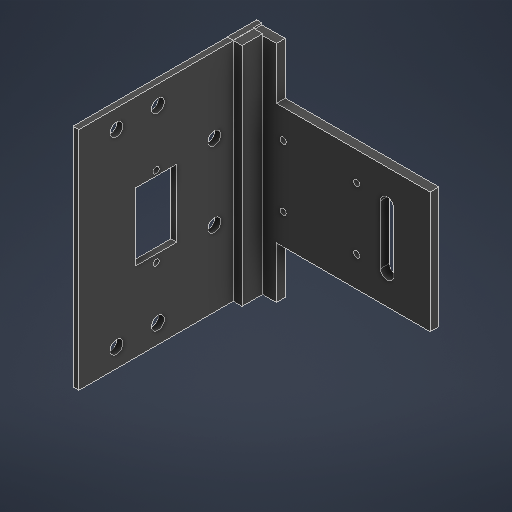
# Autodesk Inventor part: cameramount
Saved by Autodesk Inventor 2027 (Build 310192000, 192)
## iProperties
Created: 2026-06-30
Part Number: cameramount
Material: Generic
Document SubType Name: Modeling
Designer: uchiha
Density: 1 g/cm^3
Appearance: Default
Author: uchiha
Autodesk Inventor part; units mm, degrees
sketch "Sketch1" plane through (0, 0, 0) normal (1, 0, 0) x (0, 1, 0)
  circle A0 centre (-12.8712, -19.8017) radius 2.1703
  circle A1 centre (-32.0775, -0.5955) radius 2.1703
  circle A2 centre (31.9433, -0.5955) radius 2.1703
  circle A3 centre (31.9433, 13.4891) radius 2.1703
  circle A4 centre (-32.0775, 13.4891) radius 2.1703
  circle A5 centre (12.7371, -19.8017) radius 2.1703
  line L0 (38.3454, 26.2933) -> (38.3454, -26.2038)
  line L1 (-38.4796, 26.2933) -> (38.3454, 26.2933)
  line L2 (-38.4796, 26.2933) -> (-38.4796, -26.2038)
  line L3 (38.3454, -26.2038) -> (-38.4796, -26.2038)
  circle A6 centre (-32.0775, 13.4891) radius 2.1703
  circle A7 centre (-32.0775, -0.5955) radius 2.1703
  line L4 (11.5, -7) -> (-11.5, -7)
  line L5 (-11.5, -7) -> (-11.5, 7)
  line L6 (-11.5, 7) -> (11.5, 7)
  line L7 (11.5, 7) -> (11.5, -7)
  line L8 (11.5, -7) -> (-11.5, 7) construction
  line L9 (-11.5, -7) -> (11.5, 7) construction
  circle A8 centre (13.2, 0) radius 1
  circle A9 centre (-14, 0) radius 1
  point P0 (0, 0)
  point P1 (-11.5, 0)
  dimension "d26" = 23
  dimension "d27" = 14
  dimension "d28" = 27.2
  dimension "d29" = 2
  dimension "d30" = 2.5
  constraints: 20 end point, 10 centre point, 3 midpoint, 2 parallel, 1 equal radius, 1 horizontal, 1 perpendicular
  measures "d26" distance of L5.end L6.end
  measures "d27" distance of L4.end L5.end
  measures "d28" distance of A8.centre A9.centre
  measures "d29" diameter of A8
  measures "d30" distance of point (-11.5, 0) A9.centre
ref_plane "Work Plane6" through (0, -38.4796, -26.2038) normal (0, 0, -1) x (-1, 0, 0)
sketch "Sketch3" plane through (0, -38.4796, -26.2038) normal (0, 0, -1) x (-1, 0, 0)
  line L0 (0, 76.825) -> (-3, 76.825) projected
  line L1 (0, 0) -> (-3, 0) projected
  line L2 (-3, 76.825) -> (0, 76.825)
  line L3 (0, 76.825) -> (0, 0)
  line L4 (0, 0) -> (-3, 0)
  line L5 (-3, 0) -> (-3, 76.825)
  line L6 (0, 0) -> (0, 76.825) projected
  line L7 (-3, 0) -> (-3, 76.825) projected
  line L8 (0.01, -0.01) -> (0.01, 76.835)
  line L9 (0.01, 76.835) -> (-3.01, 76.835)
  line L10 (-3.01, 76.835) -> (-3.01, -0.01)
  line L11 (-3.01, -0.01) -> (0.01, -0.01)
  point P0 (0, 38.4796)
  dimension "d3" = 0.01
  constraints: 16 end point, 4 parallel, 2 perpendicular, 1 horizontal, 3 other
  measures "d3" distance between parallel lines of L3 L8
extrude "Extrusion2" add sketch "Sketch3" along normal blind 10 contours L3 L1 L5 L0
ref_plane "Work Plane3" through (0, 0, 0) normal (-1, 0, 0) x (0, 0, 1)
sketch "Sketch4" plane through (0, 0, 0) normal (-1, 0, 0) x (0, 0, 1)
  line L0 (26.2933, -38.4796) -> (-36.2038, -38.4796) projected
  line L1 (-36.2038, 38.422) -> (-33.2038, 38.422)
  line L2 (-33.2038, 38.422) -> (-33.2038, -38.4796)
  line L3 (-33.2038, -38.4796) -> (-36.2038, -38.4796)
  line L4 (-36.2038, -38.4796) -> (-36.2038, 38.422)
  line L5 (-36.2038, 38.3454) -> (-36.2038, -38.4796) projected
  point P0 (0, 0)
  dimension "d8" = 3
  constraints: 8 end point, 2 parallel, 1 collinear, 1 horizontal, 1 perpendicular, 1 point on line
  measures "d8" distance between parallel lines of L4 L2
extrude "Extrusion3" add sketch "Sketch4" against normal blind 60
ref_plane "Work Plane1" through (0, -38.4796, -36.2038) normal (0, 0, -1) x (-1, 0, 0)
ref_plane "Work Plane4" through (0, -38.4796, -36.2038) normal (0, 0, -1) x (-1, 0, 0)
sketch "Sketch6" plane through (0, -38.4796, -36.2038) normal (0, 0, -1) x (-1, 0, 0)
  line L0 (0, 38.4796) -> (-60, 38.4508)
  line L1 (-60, 0) -> (-60, 76.9016) projected
  line L2 (-30, 76.2766) -> (-30, 0)
  line L3 (-43.0944, 47.6588) -> (-43.0944, 27.6588)
  arc A0 (-47.5944, 27.6588) -> (-43.0944, 27.6588) centre (-45.3444, 27.6588) ccw
  line L4 (-47.5944, 27.6588) -> (-47.5944, 47.6588)
  arc A1 (-43.0944, 47.6588) -> (-47.5944, 47.6588) centre (-45.3444, 47.6588) ccw
  circle A2 centre (-35, 27.8243) radius 1
  circle A3 centre (-10, 27.8243) radius 1
  circle A4 centre (-35, 48.8243) radius 1
  circle A5 centre (-10, 48.8243) radius 1
  line L5 (-57.8444, 58.6588) -> (-57.8444, 17.5214)
  line L6 (-57.8444, 17.5214) -> (-2.3444, 17.5214)
  line L7 (-2.3444, 17.5214) -> (-2.3444, 58.6588)
  line L8 (-2.3444, 58.6588) -> (-57.8444, 58.6588)
  line L9 (-57.8444, 58.6588) -> (-60, 58.6588)
  line L10 (-2.3444, 58.6588) -> (0, 58.6588)
  line L11 (0, 58.6588) -> (0, 17.5214)
  line L12 (0, 17.5214) -> (-2.3444, 17.5214)
  line L13 (-57.8444, 17.5214) -> (-60, 17.5214)
  line L14 (0, 0) -> (-60, 0) projected
  line L15 (-7.6908, 17.5214) -> (-60, 17.5214)
  line L16 (-60, 17.5214) -> (-60, 0)
  line L17 (-60, 0) -> (-7.6908, 0)
  line L18 (-7.6908, 0) -> (-7.6908, 17.5214)
  line L19 (-7.6908, 76.2766) -> (-60, 76.2766)
  line L20 (-60, 76.2766) -> (-60, 58.6588)
  line L21 (-60, 58.6588) -> (-7.6908, 58.6588)
  line L22 (-7.6908, 58.6588) -> (-7.6908, 76.2766)
  point P0 (0, 76.9016)
  point P1 (-57.8444, 34.2959)
  dimension "d12" = 25
  dimension "d13" = 35
  dimension "d14" = 35
  dimension "d15" = 25
  constraints: 42 end point, 6 centre point, 6 point on line, 5 perpendicular, 4 parallel, 4 point on circle, 2 horizontal, 1 midpoint
  measures "d12" distance of A5.centre A4.centre
  measures "d13" distance from line of L11 A4.centre
  measures "d14" distance from line of L11 A2.centre
  measures "d15" distance of A3.centre A2.centre
extrude "Extrusion4" cut sketch "Sketch6" against normal blind 60 contours L3 A0 L4 L0 | L0 L4 A1 L3 | L8 L9 L1 L19 L2 | L2 L19 L22 L8 | L6 L18 L14 L2 | L2 L14 L1 L13 L6 | A2 | A3 | A4 | A5
sketch "Sketch7" plane through (0, -38.4796, -36.2038) normal (0, 0, -1) x (-1, 0, 0)
  point P0 (0, 38.4796)
extrude "Extrusion7" add sketch "Sketch1" against normal blind 2
ref_plane "Work Plane7" through (0, 38.422, -36.2038) normal (-1, 0, 0) x (0, 0, 1)
sketch "Sketch9" plane through (0, 38.422, -36.2038) normal (-1, 0, 0) x (0, 0, 1)
  line L0 (0, -76.9016) -> (0, 0) projected
  line L1 (0, 0) -> (10, 0)
  line L2 (10, 0) -> (10, -76.9016)
  line L3 (10, -76.9016) -> (0, -76.9016)
  line L4 (0, -76.9016) -> (0, 0)
  point P0 (36.2038, -38.422)
  constraints: 8 end point, 2 parallel, 1 horizontal, 1 perpendicular
extrude "Extrusion8" add sketch "Sketch9" along normal blind 2
sketch "Sketch10" plane through (60, 0, 0) normal (1, 0, 0) x (0, 0, -1)
  line L0 (36.2038, 38.422) -> (33.2038, 38.422) projected
  line L1 (33.2038, 37.797) -> (36.2038, 37.797) projected
  line L2 (33.2038, 38.422) -> (36.2038, 38.422)
  line L3 (36.2038, 38.422) -> (36.2038, 37.797)
  line L4 (36.2038, 37.797) -> (33.2038, 37.797)
  line L5 (33.2038, 37.797) -> (33.2038, 38.422)
  point P0 (0, 0)
  constraints: 8 end point, 2 parallel, 1 horizontal, 1 perpendicular
extrude "Extrusion9" cut sketch "Sketch10" against normal blind 60.25
body "Solid1"
